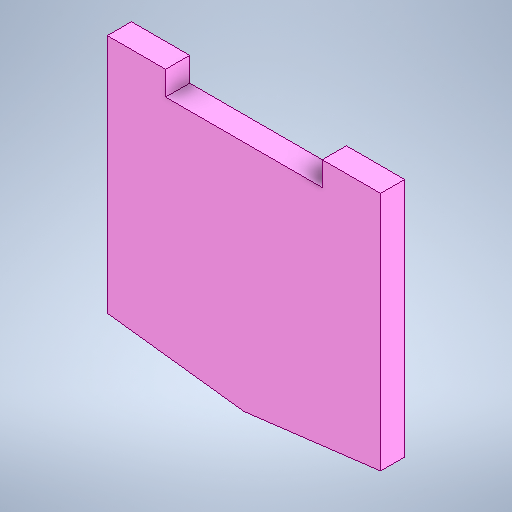
# Autodesk Inventor part: A
Saved by Autodesk Inventor 2025.3 (Build 293356030, 356C)
## iProperties
Created: 2025-07-09
Part Number: A
Material: Generic
Document SubType Name: Modeling
Designer: jv
Density: 1 g/cm^3
Appearance: Default(2)
Author: jv
Autodesk Inventor part; units mm, degrees
ref_plane "YZ Plane" through (0, 0, 0) normal (1, 0, 0) x (0, 1, 0)
ref_plane "XZ Plane" through (0, 0, 0) normal (0, 1, 0) x (-1, 0, 0)
ref_plane "XY Plane" through (0, 0, 0) normal (0, 0, 1) x (1, 0, 0)
sketch "Sketch1" plane through (0, 0, 0) normal (0, 0, 1) x (1, 0, 0)
  line L0 (-17, 16) -> (17, 16)
  line L1 (17, 16) -> (17, -16)
  line L2 (17, -16) -> (-17, -16)
  line L3 (-17, -16) -> (-17, 16)
  line L4 (-9.75, 16) -> (9.75, 16)
  line L5 (9.75, 16) -> (9.75, 13)
  line L6 (9.75, 13) -> (-9.75, 13)
  line L7 (-9.75, 13) -> (-9.75, 16)
  line L8 (0, -16) -> (0, -13.92)
  line L9 (17, -13.92) -> (0, -16)
  line L10 (0, -16) -> (-17, -13.92)
  point P0 (0, 0)
  point P1 (17, 0)
  point P2 (0, 16)
  point P3 (9.75, 16)
  dimension "d0" = 34
  dimension "d1" = 32
  dimension "d3" = 2.08
  dimension "d6" = 19.5
  dimension "d7" = 3
  constraints: 22 end point, 4 midpoint, 4 parallel, 3 point on line, 2 horizontal, 2 perpendicular, 1 horizontal alignment, 1 vertical, 1 vertical alignment
  measures "d0" distance of L0.start L0.end
  measures "d1" distance of L0.end L1.end
  measures "d3" distance of L8.start L8.end
  measures "d6" distance of L5.end L6.end
  measures "d7" distance of L4.end L5.end
extrude "Extrusion1" add sketch "Sketch1" along normal mid plane 3 contours L0 L7 L6 L5 L1 L9 L10 L3
body "Solid1"
